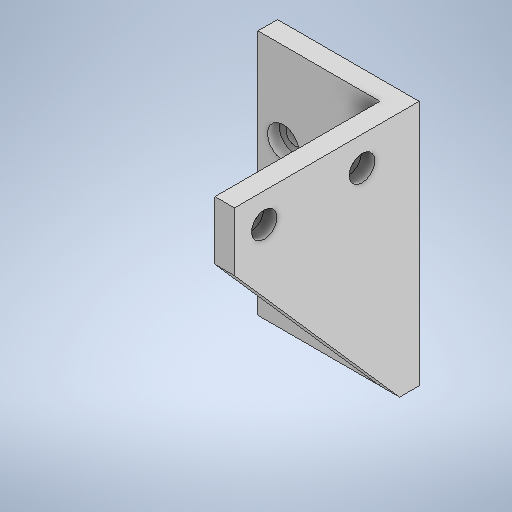
# Autodesk Inventor part: TS_Adapter_Greifer_int
Saved by Autodesk Inventor 2025.2 (Build 292293000, 293)
## iProperties
Created: 2025-06-16
Part Number: TS_Adapter_Greifer_int
Material: Generisch
Document SubType Name: Modeling
Designer: tino
Density: 1 g/cm^3
Appearance: Vorgabe
Author: tino
Autodesk Inventor part; units mm, degrees
ref_plane "YZ Plane" through (0, 0, 0) normal (1, 0, 0) x (0, 1, 0)
ref_plane "XZ Plane" through (0, 0, 0) normal (0, 1, 0) x (-1, 0, 0)
ref_plane "XY Plane" through (0, 0, 0) normal (0, 0, 1) x (1, 0, 0)
sketch "Skizze1" plane through (0, 0, 0) normal (0, 0, 1) x (1, 0, 0)
  line L0 (-19.75, 23.6) -> (19.75, 23.6)
  line L1 (19.75, 23.6) -> (19.75, -23.6)
  line L2 (19.75, -23.6) -> (-19.75, -23.6)
  line L3 (-19.75, -23.6) -> (-19.75, 23.6)
  line L4 (0, 33.04) -> (0, -33.04) projected
  line L5 (-27.65, 0) -> (27.65, 0) projected
  point P0 (0, 0)
  dimension "d0" = 39.5
  dimension "d1" = 47.2
  dimension "d46" = 19.75
  dimension "d47" = 23.6
  constraints: 8 end point, 2 parallel, 1 horizontal, 1 perpendicular
  measures "d0" distance of L1.end L2.end
  measures "d1" distance of L2.end L0.start
  measures "d46" distance between parallel lines of L3 L4
  measures "d47" distance between parallel lines of L5 L2
extrude "Extrusion1" add sketch "Skizze1" along normal blind 63
sketch "Skizze2" plane through (0, 0, 63) normal (0, 0, 1) x (1, 0, 0)
  line L0 (-19.75, -23.6) -> (19.75, -23.6) projected
  line L1 (-19.75, -23.6) -> (14.75, -23.6)
  line L2 (14.75, -23.6) -> (14.75, 18.6)
  line L3 (14.75, 18.6) -> (-19.75, 18.6)
  line L4 (-19.75, 18.6) -> (-19.75, -23.6)
  line L5 (-19.75, 23.6) -> (-19.75, -23.6) projected
  line L6 (19.75, 23.6) -> (-19.75, 23.6) projected
  point P0 (0, 0)
  point P1 (14.75, -23.6)
  dimension "d4" = 34.5
  dimension "d6" = 5
  constraints: 8 end point, 2 parallel, 1 collinear, 1 horizontal, 1 perpendicular, 1 point on line
  measures "d4" distance of L2.end L3.end
  measures "d6" distance between parallel lines of L6 L3
extrude "Extrusion2" cut sketch "Skizze2" against normal through all
sketch "Skizze4" plane through (-19.75, 18.6, 0) normal (0, 1, 0) x (1, 0, 0)
  line L0 (39.5, -63) -> (0, -63) projected
  line L1 (39.5, 0) -> (0, 0) projected
  line L2 (0, -63) -> (34.5, -63) construction
  line L3 (19.75, -63) -> (19.75, 0)
  line L4 (39.5, 0) -> (39.5, -63) construction
  line L5 (0, 0) -> (0, -63) projected
  point P0 (29.75, -41.5)
  point P1 (9.75, -41.5)
  point P2 (29.75, -21.5)
  point P3 (9.75, -21.5)
  dimension "d9" = 20
  dimension "d14" = 19.75
  dimension "d16" = 10
  dimension "d17" = 63
  dimension "d63" = 20
  dimension "d64" = 21.5
  dimension "d65" = 39.5
  constraints: 2 end point, 2 horizontal alignment, 2 vertical alignment, 1 midpoint, 1 point on line
  measures "d9" distance of point (29.75, -21.5) point (29.75, -41.5)
  measures "d14" distance between parallel lines of L4 L3
  measures "d16" distance from line of point (9.75, -21.5) L3
  measures "d17" distance of L1.end L0.end
  measures "d63" distance of point (29.75, -41.5) point (9.75, -41.5)
  measures "d64" distance from line of L1 point (9.75, -21.5)
  measures "d65" distance between parallel lines of L4 L5
hole "Bohrung1" at (10, 18.6, 41.5) at (-10, 18.6, 41.5) at (10, 18.6, 21.5) at (-10, 18.6, 21.5) direction (0, 1, 0) diameter 4.5 end through all counterbore diameter 8 counterbore depth 3
sketch "Skizze5" plane through (19.75, -23.6, 0) normal (1, 0, 0) x (0, 0, -1)
  line L0 (-63, 42.2) -> (0, 42.2) projected
  line L1 (-63, 0) -> (-63, 47.2) projected
  point P0 (0, 23.6)
  point P1 (-55.5, 7.6)
  point P2 (-55.5, 32.6)
  dimension "d36" = 25
  dimension "d37" = 9.6
  dimension "d38" = 7.5
  constraints: 1 vertical alignment
  measures "d36" distance of point (-55.5, 32.6) point (-55.5, 7.6)
  measures "d37" distance from line of L0 point (-55.5, 32.6)
  measures "d38" distance from line of L1 point (-55.5, 7.6)
hole "Bohrung3" at (19.75, -16, 55.5) at (19.75, 9, 55.5) direction (-1, 0, 0) diameter 3.4 depth 5 counterbore diameter 6.5 counterbore depth 3.4
sketch "Skizze6" plane through (-19.75, 23.6, 0) normal (0, 1, 0) x (1, 0, 0)
  line L0 (39.5, -63) -> (0, -63) projected
  line L1 (39.5, 0) -> (0, 0) projected
  line L2 (19.75, 12.6) -> (19.75, -75.6) projected
  point P0 (19.75, 0)
  point P1 (19.75, -44)
  point P2 (19.75, -19)
  dimension "d48" = 25
  dimension "d49" = 63
  dimension "d50" = 19
  constraints: 1 point on line, 1 vertical alignment
  measures "d48" distance of point (19.75, -19) point (19.75, -44)
  measures "d49" distance between parallel lines of L0 L1
  measures "d50" distance from line of L1 point (19.75, -19)
hole "Bohrung4" at (0, 23.6, 44) at (0, 23.6, 19) direction (0, -1, 0) diameter 5 depth 2.5
sketch "Skizze7" plane through (19.75, -23.6, 0) normal (1, 0, 0) x (0, 0, -1)
  line L0 (0, 0) -> (0, 42.2) projected
  line L1 (-48, 0) -> (0, 42.2)
  line L2 (0, 0) -> (-63, 0) projected
  line L3 (0, 47.2) -> (-63, 47.2) projected
  line L4 (-63, 0) -> (-63, 47.2) projected
  point P0 (0, 23.6)
  dimension "d58" = 5
  dimension "d59" = 15
  constraints: 2 end point, 1 point on line
  measures "d58" distance from line of L3 L0.end
  measures "d59" distance from line of L4 L1.start
extrude "Extrusion3" cut sketch "Skizze7" against normal through all
sketch "Skizze8" plane through (-19.75, 18.6, 63) normal (0, -1, 0) x (1, 0, 0)
  line L0 (34.5, -63) -> (0, -63) projected
  line L1 (0, 0) -> (3.3, 0)
  line L2 (3.3, 0) -> (3.3, -63)
  line L3 (3.3, -63) -> (0, -63)
  line L4 (0, -63) -> (0, 0)
  point P0 (19.75, -63)
  point P1 (0, -63)
  dimension "d66" = 3.3
  constraints: 8 end point, 2 parallel, 1 horizontal, 1 perpendicular, 1 point on line
  measures "d66" distance between parallel lines of L4 L2
extrude "Extrusion4" cut sketch "Skizze8" against normal through all
equation "\"d46\" = 0.5 * d0"
equation "\"d47\" = 0.5 * d1"
equation "\"d6\" = d5"
equation "\"d16\" = 0.5 * d12"
equation "\"d50\" = -0.5 * d48 + 0.5 * d49"
equation "\"d5\" = 5"
equation "\"d12\" = 20"
